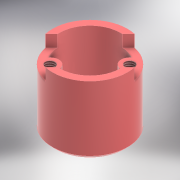
# Autodesk Inventor part: BRAÇO ROBÓTICO - Garra A4b
Saved by Autodesk Inventor 2021 (Build 250183000, 183)
## iProperties
Created: 2020-09-26
Part Number: BRAÇO ROBÓTICO - Garra A4b
Material: Plástico PC/ABS
Document SubType Name: Modeling
Designer: Araújo, I.
Mass: 1.161 g
Surface Area: 32.7291 cm^2
Volume: 3.24963 cm^3
Density: 0.357273 g/cm^3
Appearance: Liso - Branco
Author: Araújo, I.
## iProperties of the stored document _3DPrint.ipt
Created: 2020-11-26
Part Number: _3DPrint
Material: Genérico
Document SubType Name: Modeling
Designer: Araújo, I.
Mass: 3.29039 g
Surface Area: 32.422 cm^2
Volume: 3.29039 cm^3
Density: 1 g/cm^3
Appearance: Padrão
Author: Araújo, I.
Autodesk Inventor part; units mm, degrees
ref_plane "YZ Plane" through (0, 0, 0) normal (1, 0, 0) x (0, 1, 0)
ref_plane "XZ Plane" through (0, 0, 0) normal (0, 1, 0) x (-1, 0, 0)
ref_plane "XY Plane" through (0, 0, 0) normal (0, 0, 1) x (1, 0, 0)
sketch "Esboço1" plane through (0, 0, 0) normal (0, 0, 1) x (1, 0, 0)
  line L0 (-9, 20) -> (-9, 4)
  line L1 (-9, 4) -> (0, 4)
  line L2 (0, 4) -> (0, 0)
  line L3 (0, 0) -> (-10, 0)
  line L4 (-11, 1) -> (-11, 20)
  line L5 (-11, 1) -> (-10, 0)
  line L6 (-11, 20) -> (-9, 20)
  dimension "d0" = 18
  dimension "d1" = 2
  dimension "d2" = 4
  dimension "d10" = 45
  dimension "d11" = 1
  dimension "d30" = 20
  constraints: 14 end point, 5 perpendicular, 1 coincident, 1 vertical
  measures "d0" diameter of L0 L2
  measures "d1" distance between parallel lines of L0 L4
  measures "d2" distance between parallel lines of L3 L1
  measures "d10" angle of L3 L5
  measures "d11" distance from line of L4.start L3
  measures "d30" distance between parallel lines of L3 L6
revolve "Revolução1" add sketch "Esboço1" angle 360 about axis through (0, 4, 0) along (0, -1, 0)
sketch "Esboço2" plane through (0, 4, 0) normal (0, 1, 0) x (1, 0, 0)
  circle A0 centre (0, 0) radius 3.5
  circle A1 centre (0, 0) radius 6.35 construction
  circle A2 centre (0, 6.35) radius 1.25
  circle A3 centre (0, -6.35) radius 1.25
  circle A4 centre (-6.35, 0) radius 1.25
  circle A5 centre (6.35, 0) radius 1.25
  circle A6 centre (0, 6.35) radius 2.5
  dimension "d12" = 7
  dimension "d13" = 12.7
  dimension "d14" = 2.5
  dimension "d48" = 5
  constraints: 7 centre point, 4 point on circle, 3 equal radius, 2 coincident, 2 horizontal alignment, 2 vertical alignment, 1 concentric
  measures "d12" diameter of A0
  measures "d13" diameter of A1
  measures "d14" diameter of A2
  measures "d48" diameter of A6
extrude "Extrusão1" cut sketch "Esboço2" against normal through all contours A0 | A2 | A3 | A4 | A5
sketch "Esboço5" plane through (0, 20, 0) normal (0, 1, 0) x (1, 0, 0)
  circle A0 centre (0, 0) radius 9 projected
  arc A1 (-4.3758, -7.8646) -> (-7.8646, -4.3758) centre (-5.8336, -5.8336) ccw
  line L0 (-15.4, 0) -> (15.4, 0) projected
  circle A2 centre (0, 0) radius 8.25 construction
  arc A3 (4.3758, 7.8646) -> (7.8646, 4.3758) centre (5.8336, 5.8336) ccw
  line L1 (-5.8336, -5.8336) -> (5.8336, 5.8336) construction
  dimension "d32" = 2.5
  dimension "d49" = 45
  dimension "d50" = 16.5
  constraints: 10 point on circle, 3 centre point, 2 end point, 1 coincident, 1 equal radius, 1 midpoint
  measures "d32" radius of A1
  measures "d49" angle of L1 L0
  measures "d50" diameter of A2
extrude "Extrusão4" add sketch "Esboço5" against normal up to surface (16 mm away) contours A3 A0 | A0 A1
sketch "Esboço7" plane through (0, 20, 0) normal (0, 1, 0) x (1, 0, 0)
  arc A0 (-4.3758, -7.8646) -> (-7.8646, -4.3758) centre (-5.8336, -5.8336) ccw projected
  arc A1 (4.3758, 7.8646) -> (7.8646, 4.3758) centre (5.8336, 5.8336) ccw projected
  point P0 (0, 0)
hole "Furo1" at (-5.8336, 20, 5.8336) at (5.8336, 20, -5.8336) direction (0, -1, 0) diameter 2.85 depth 16 thread size "M3.5x0.6" class "6H" standard "ANSI Metric M Profile"
sketch "Esboço6" plane through (0, 20, 0) normal (0, 1, 0) x (1, 0, 0)
  circle A0 centre (0, 0) radius 11 projected
  line L0 (2.2766, 10.7618) -> (-10.7618, -2.2766)
  line L1 (10.7618, 2.2766) -> (-2.2766, -10.7618)
  circle A1 centre (0, 0) radius 11 projected
  line L2 (-5.8336, -5.8336) -> (5.8336, 5.8336) construction
  circle A2 centre (-5.8336, -5.8336) radius 1.425 projected
  circle A3 centre (5.8336, 5.8336) radius 1.425 projected
  point P0 (-2.2766, -10.7618)
  dimension "d45" = 12
  constraints: 6 end point, 4 point on circle, 3 parallel, 2 coincident
  measures "d45" distance between parallel lines of L0 L1
extrude "Extrusão5" cut sketch "Esboço6" against normal blind 3.5 contours L1 A0 L0 | A2 | A3
